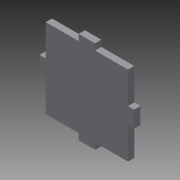
# Autodesk Inventor part: back
Saved by Autodesk Inventor 2015 SP1 (Build 190203100, 203)
## iProperties
Created: 2016-04-13
Part Number: back
Material: Generic
Document SubType Name: Modeling
Designer: tuttlem
Density: 1 g/cm^3
Appearance: Default
Author: tuttlem
Autodesk Inventor part; units mm, degrees
ref_plane "YZ Plane" through (0, 0, 0) normal (1, 0, 0) x (0, 1, 0)
ref_plane "XZ Plane" through (0, 0, 0) normal (0, 1, 0) x (-1, 0, 0)
ref_plane "XY Plane" through (0, 0, 0) normal (0, 0, 1) x (1, 0, 0)
sketch "Sketch1" plane through (0, 0, 0) normal (0, 0, 1) x (1, 0, 0)
  line L0 (0, 0) -> (19.05, 0) projected
  line L1 (19.05, 0) -> (19.05, 4.826) projected
  line L2 (0, 4.826) -> (19.05, 4.826) projected
  line L3 (0, 0) -> (0, 4.826) projected
  line L4 (19.05, 0) -> (31.75, 0) projected
  line L5 (31.75, 0) -> (31.75, 4.826) projected
  line L6 (19.05, 4.826) -> (31.75, 4.826) projected
  line L7 (19.05, 0) -> (19.05, 4.826) projected
  line L8 (31.75, 0) -> (50.8, 0) projected
  line L9 (50.8, 0) -> (50.8, 4.826) projected
  line L10 (31.75, 4.826) -> (50.8, 4.826) projected
  line L11 (31.75, 0) -> (31.75, 4.826) projected
  line L12 (50.8, 4.826) -> (55.626, 4.826) projected
  line L13 (50.8, 0) -> (50.8, 4.826) projected
  line L14 (55.626, 0) -> (50.8, 0) projected
  line L15 (55.626, 4.826) -> (55.626, 0) projected
  line L16 (50.8, -61.5142) -> (55.626, -61.5142) projected
  line L17 (50.8, -66.3402) -> (50.8, -61.5142) projected
  line L18 (55.626, -66.3402) -> (50.8, -66.3402) projected
  line L19 (55.626, -61.5142) -> (55.626, -66.3402) projected
  line L20 (31.75, -66.3402) -> (50.8, -66.3402) projected
  line L21 (50.8, -66.3402) -> (50.8, -61.5142) projected
  line L22 (31.75, -61.5142) -> (50.8, -61.5142) projected
  line L23 (31.75, -66.3402) -> (31.75, -61.5142) projected
  line L24 (38.1, -66.3402) -> (38.1, -61.5142) projected
  line L25 (25.4, -61.5142) -> (31.75, -61.5142) projected
  line L26 (0, -66.3402) -> (25.4, -66.3402) projected
  line L27 (0, -61.5142) -> (25.4, -61.5142) projected
  line L28 (0, -66.3402) -> (0, -61.5142) projected
  line L29 (-4.826, 7.366) -> (-4.826, -68.834) projected
  line L30 (-4.826, -68.834) -> (0, -68.834) projected
  line L31 (0, 7.366) -> (0, -68.834) projected
  line L32 (-4.826, 7.366) -> (0, 7.366) projected
  line L33 (-4.826, -37.084) -> (-4.826, -24.384) projected
  line L34 (-4.826, -37.084) -> (0, -37.084) projected
  line L35 (0, -24.384) -> (0, -37.084) projected
  line L36 (-4.826, -24.384) -> (0, -24.384) projected
  line L37 (31.75, 4.826) -> (19.05, 4.826)
  line L38 (19.05, 4.826) -> (19.05, 0)
  line L39 (19.05, 0) -> (31.75, 0)
  line L40 (31.75, 0) -> (31.75, 4.826)
  line L41 (31.75, -61.5142) -> (19.05, -61.5142)
  line L42 (0, -24.384) -> (-4.826, -24.384)
  line L43 (-4.826, -24.384) -> (-4.826, -37.084)
  line L44 (-4.826, -37.084) -> (0, -37.084)
  line L45 (0, -37.084) -> (0, -24.384)
  line L46 (50.8, 0) -> (0, 0)
  line L47 (0, 0) -> (0, -61.5142)
  line L48 (0, -61.5142) -> (50.8, -61.5142)
  line L49 (50.8, -61.5142) -> (50.8, 0)
  line L50 (31.75, -66.3402) -> (19.05, -66.3402)
  line L51 (19.05, -66.3402) -> (19.05, -61.5142)
  line L52 (19.05, -61.5142) -> (31.75, -61.5142)
  line L53 (31.75, -61.5142) -> (31.75, -66.3402)
  line L54 (31.75, 0) -> (19.05, 0)
  line L55 (19.05, 0) -> (19.05, 4.826)
  line L56 (19.05, 4.826) -> (31.75, 4.826)
  line L57 (31.75, 4.826) -> (31.75, 0)
  line L58 (50.8, -24.384) -> (55.626, -24.384)
  line L59 (55.626, -24.384) -> (55.626, -37.084)
  line L60 (55.626, -37.084) -> (50.8, -37.084)
  line L61 (50.8, -37.084) -> (50.8, -24.384)
  point P0 (50.8, -37.084)
  constraints: 50 end point, 12 parallel, 7 horizontal, 6 perpendicular, 4 point on line
ref_plane "Work Plane2" through (0, 0, 0) normal (0, 0, 1) x (1, 0, 0)
sketch "Sketch2" plane through (0, 0, 0) normal (0, 0, 1) x (1, 0, 0)
  point P0 (0, 0)
ref_plane "Work Plane1" through (0, 0, -4.826) normal (0, 0, -1) x (-1, 0, 0)
sketch "Sketch3" plane through (0, 0, -4.826) normal (0, 0, -1) x (-1, 0, 0)
  point P0 (0, 0)
extrude "Extrusion2" add sketch "Sketch1" against normal blind 4.826 contours L0 L4 L8 L49 L22 L25 L27 L31 | L1 L6 L5 L4 | L31 L34 L29 L36 | L58 L59 L60 L49 | L27 L25 L23 L50 L26 L51
body "Solid2"
